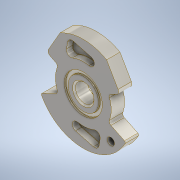
# Autodesk Inventor part: Part005. Frontal Faucet Core
Saved by Autodesk Inventor 2022.2 (Build 262287010, 287A)
## iProperties
Created: 2022-11-29
Part Number: Part005. Frontal Faucet Core
Material: Stainless Steel
Document SubType Name: Modeling
Designer: User
Mass: 160.563 g
Surface Area: 77.5804 cm^2
Volume: 20.0704 cm^3
Density: 8 g/cm^3
Appearance: Titanium - Polished
Author: User
Autodesk Inventor part; units mm, degrees
ref_plane "YZ Plane" through (0, 0, 0) normal (1, 0, 0) x (0, 1, 0)
ref_plane "XZ Plane" through (0, 0, 0) normal (0, 1, 0) x (-1, 0, 0)
sketch "Sketch1" plane through (0, 0, 0) normal (0, 0, 1) x (1, 0, 0)
  arc A0 (-28.473878, -15.0359) -> (28.473878, -15.0359) centre (0, 0) ccw
  arc A1 (-17.077087, -8.329052) -> (-17.077087, 8.329052) centre (0, 0) ccw construction
  line L0 (-18.788881, 9.163949) -> (-22.595928, 11.02077)
  line L1 (-23.665064, 14.517756) -> (-15.871417, 28.016747)
  line L2 (-18.788881, -9.163949) -> (-28.027967, -13.670153)
  arc A2 (-15.871417, 28.016747) -> (-28.941168, -14.115551) centre (0, 0) ccw construction
  arc A3 (-17.792706, 6.664803) -> (-17.792706, -6.664803) centre (0, 0) ccw
  line L3 (0, -45.08) -> (0, 45.08) construction
  line L4 (-69.758488, 0) -> (68.933664, 0) construction
  arc A4 (-17.792706, 6.664803) -> (-18.788881, 9.163949) centre (-19.665623, 7.366361) ccw
  arc A5 (-18.788881, -9.163949) -> (-17.792706, -6.664803) centre (-19.665623, -7.366361) ccw
  arc A6 (-28.027967, -13.670153) -> (-28.473878, -15.0359) centre (-27.589596, -14.568947) ccw
  arc A7 (-23.665064, 14.517756) -> (-22.595928, 11.02077) centre (-21.5, 13.267756) ccw
  arc A8 (17.077087, 8.329052) -> (17.077087, -8.329052) centre (0, 0) ccw construction
  line L5 (18.788881, 9.163949) -> (22.595928, 11.02077)
  line L6 (23.665064, 14.517756) -> (15.871417, 28.016747)
  line L7 (18.788881, -9.163949) -> (28.027967, -13.670153)
  arc A9 (28.941168, -14.115551) -> (32.2, 0) centre (0, 0) ccw construction
  arc A10 (17.792706, -6.664803) -> (17.792706, 6.664803) centre (0, 0) ccw
  line L8 (69.758488, 0) -> (-68.933664, 0) construction
  arc A11 (18.788881, 9.163949) -> (17.792706, 6.664803) centre (19.665623, 7.366361) ccw
  arc A12 (17.792706, -6.664803) -> (18.788881, -9.163949) centre (19.665623, -7.366361) ccw
  arc A13 (28.473878, -15.0359) -> (28.027967, -13.670153) centre (27.589596, -14.568947) ccw
  arc A14 (22.595928, 11.02077) -> (23.665064, 14.517756) centre (21.5, 13.267756) ccw
  arc A15 (32.2, 0) -> (15.871417, 28.016747) centre (0, 0) ccw construction
  arc A16 (32.2, 0) -> (15.871417, 28.016747) centre (0, 0) ccw construction
  arc A17 (28.473878, -15.0359) -> (32.2, 0) centre (0, 0) ccw construction
  arc A18 (15.871417, 28.016747) -> (-15.871417, 28.016747) centre (0, 0) ccw
  circle A19 centre (0, 0) radius 6.3
  dimension "d0" = 64.4
  dimension "d1" = 38
  dimension "d2" = 26
  dimension "d3" = 52
  dimension "d4" = 30
  dimension "d5" = 2
  dimension "d6" = 1
  dimension "d7" = 2.5
  dimension "d8" = 48
  dimension "d9" = 12.6
  constraints: 43 point on circle, 20 centre point, 18 symmetric about line, 14 end point, 9 point on line, 8 tangent, 4 coincident, 1 equal radius, 7 other
  measures "d0" diameter of A0
  measures "d1" diameter of A1
  measures "d2" angle of L4 L2
  measures "d3" angle of L2 L0
  measures "d4" angle of L3 L1
  measures "d5" radius of A4
  measures "d6" radius of A6
  measures "d7" radius of A7
  measures "d9" diameter of A19
extrude "Extrusion1" add sketch "Sketch1" along normal blind 9.1
sketch "Sketch2" plane through (0, 0, 9.1) normal (0, 0, 1) x (1, 0, 0)
  arc A0 (-28.027967, -13.670153) -> (-28.473878, -15.0359) centre (-27.589596, -14.568947) ccw
  arc A1 (-28.473878, -15.0359) -> (28.473878, -15.0359) centre (0, 0) ccw
  arc A2 (28.473878, -15.0359) -> (28.027967, -13.670153) centre (27.589596, -14.568947) ccw
  line L0 (28.027967, -13.670153) -> (18.788881, -9.163949)
  arc A3 (17.792706, -6.664803) -> (18.788881, -9.163949) centre (19.665623, -7.366361) ccw
  arc A4 (17.792706, -6.664803) -> (17.792706, 6.664803) centre (0, 0) ccw
  arc A5 (18.788881, 9.163949) -> (17.792706, 6.664803) centre (19.665623, 7.366361) ccw
  line L1 (18.788881, 9.163949) -> (22.595928, 11.02077)
  arc A6 (22.595928, 11.02077) -> (23.665064, 14.517756) centre (21.5, 13.267756) ccw
  line L2 (23.665064, 14.517756) -> (15.871417, 28.016747)
  arc A7 (15.871417, 28.016747) -> (-15.871417, 28.016747) centre (0, 0) ccw
  line L3 (-15.871417, 28.016747) -> (-23.665064, 14.517756)
  arc A8 (-23.665064, 14.517756) -> (-22.595928, 11.02077) centre (-21.5, 13.267756) ccw
  line L4 (-22.595928, 11.02077) -> (-18.788881, 9.163949)
  arc A9 (-17.792706, 6.664803) -> (-18.788881, 9.163949) centre (-19.665623, 7.366361) ccw
  arc A10 (-17.792706, 6.664803) -> (-17.792706, -6.664803) centre (0, 0) ccw
  arc A11 (-18.788881, -9.163949) -> (-17.792706, -6.664803) centre (-19.665623, -7.366361) ccw
  line L5 (-18.788881, -9.163949) -> (-28.027967, -13.670153)
  circle A12 centre (0, 0) radius 6.3
  arc A13 (17.792706, 6.664803) -> (3.886364, 18.598284) centre (0, 0) ccw construction
  arc A14 (-11.454423, 20.812568) -> (-7.340909, 17.524584) centre (-8.5, 20.291624) ccw
  arc A15 (3.886364, 18.598284) -> (5.276457, 24.432633) centre (4.5, 21.534855) ccw
  line L6 (0, -45.08) -> (0, 45.08) construction
  line L7 (-11.454423, 20.812568) -> (-10.658601, 25.3259)
  line L8 (-6.927721, 27.702733) -> (5.276457, 24.432633)
  arc A16 (-6.927721, 27.702733) -> (-10.658601, 25.3259) centre (-7.704178, 24.804955) ccw
  arc A17 (-7.340909, 17.524584) -> (-17.792706, 6.664803) centre (0, 0) ccw construction
  arc A18 (3.886364, 18.598284) -> (-7.340909, 17.524584) centre (0, 0) ccw
  arc A19 (6.927721, -27.702733) -> (10.658601, -25.3259) centre (7.704178, -24.804955) ccw
  arc A20 (7.340909, -17.524584) -> (17.792706, -6.664803) centre (0, 0) ccw construction
  arc A21 (-17.792706, -6.664803) -> (-3.886364, -18.598284) centre (0, 0) ccw construction
  arc A22 (-3.886364, -18.598284) -> (7.340909, -17.524584) centre (0, 0) ccw
  arc A23 (11.454423, -20.812568) -> (7.340909, -17.524584) centre (8.5, -20.291624) ccw
  arc A24 (-3.886364, -18.598284) -> (-5.276457, -24.432633) centre (-4.5, -21.534855) ccw
  line L9 (11.454423, -20.812568) -> (10.658601, -25.3259)
  line L10 (6.927721, -27.702733) -> (-5.276457, -24.432633)
  dimension "d12" = 6
  dimension "d13" = 11.5
  dimension "d14" = 13
  dimension "d15" = 3
  dimension "d16" = 10
  dimension "d20" = 360
  constraints: 24 point on circle, 12 centre point, 8 end point, 6 tangent, 1 coincident, 1 equal radius, 41 other
  measures "d12" diameter of A14
  measures "d14" horizontal distance of A15.centre A14.centre
  measures "d15" radius of A16
  measures "d16" angle of L6 L7
extrude "Extrusion2" cut sketch "Sketch2" against normal blind 4.3 contours L7 A16 L8 A15 A18 A14 | L10 A24 A22 A23 L9 A19
fillet "Fillet1" radius 0.2 12 edges at (-10.3731, 17.9482, 4.8) (-11.0565, 23.0692, 4.8) (-9.3161, 27.3351, 4.8) (-0.8256, 26.0677, 4.8) (7.4183, 20.8395, 4.8) (-1.8088, 18.9137, 4.8) (-7.4183, -20.8395, 4.8) (1.8088, -18.9137, 4.8) (10.3731, -17.9482, 4.8) (11.0565, -23.0692, 4.8) (9.3161, -27.3351, 4.8) (0.8256, -26.0677, 4.8)
sketch "Sketch3" plane through (0, 0, 9.1) normal (0, 0, 1) x (1, 0, 0)
  arc A0 (6.927721, -27.702733) -> (10.658601, -25.3259) centre (7.704178, -24.804955) ccw
  line L0 (6.927721, -27.702733) -> (-5.276457, -24.432633)
  arc A1 (-3.886364, -18.598284) -> (-5.276457, -24.432633) centre (-4.5, -21.534855) ccw
  arc A2 (-3.886364, -18.598284) -> (7.340909, -17.524584) centre (0, 0) ccw
  arc A3 (11.454423, -20.812568) -> (7.340909, -17.524584) centre (8.5, -20.291624) ccw
  line L1 (11.454423, -20.812568) -> (10.658601, -25.3259)
  arc A4 (-11.454423, 20.812568) -> (-7.340909, 17.524584) centre (-8.5, 20.291624) ccw
  line L2 (-11.454423, 20.812568) -> (-10.658601, 25.3259)
  arc A5 (-6.927721, 27.702733) -> (-10.658601, 25.3259) centre (-7.704178, 24.804955) ccw
  line L3 (-6.927721, 27.702733) -> (5.276457, 24.432633)
  arc A6 (3.886364, 18.598284) -> (5.276457, 24.432633) centre (4.5, 21.534855) ccw
  arc A7 (3.886364, 18.598284) -> (-7.340909, 17.524584) centre (0, 0) ccw
  arc A8 (-28.027967, -13.670153) -> (-28.473878, -15.0359) centre (-27.589596, -14.568947) ccw
  arc A9 (-28.473878, -15.0359) -> (28.473878, -15.0359) centre (0, 0) ccw
  arc A10 (28.473878, -15.0359) -> (28.027967, -13.670153) centre (27.589596, -14.568947) ccw
  line L4 (28.027967, -13.670153) -> (18.788881, -9.163949)
  arc A11 (17.792706, -6.664803) -> (18.788881, -9.163949) centre (19.665623, -7.366361) ccw
  arc A12 (17.792706, -6.664803) -> (17.792706, 6.664803) centre (0, 0) ccw
  arc A13 (18.788881, 9.163949) -> (17.792706, 6.664803) centre (19.665623, 7.366361) ccw
  line L5 (18.788881, 9.163949) -> (22.595928, 11.02077)
  arc A14 (22.595928, 11.02077) -> (23.665064, 14.517756) centre (21.5, 13.267756) ccw
  line L6 (23.665064, 14.517756) -> (15.871417, 28.016747)
  arc A15 (15.871417, 28.016747) -> (-15.871417, 28.016747) centre (0, 0) ccw
  line L7 (-15.871417, 28.016747) -> (-23.665064, 14.517756)
  arc A16 (-23.665064, 14.517756) -> (-22.595928, 11.02077) centre (-21.5, 13.267756) ccw
  line L8 (-22.595928, 11.02077) -> (-18.788881, 9.163949)
  arc A17 (-17.792706, 6.664803) -> (-18.788881, 9.163949) centre (-19.665623, 7.366361) ccw
  arc A18 (-17.792706, 6.664803) -> (-17.792706, -6.664803) centre (0, 0) ccw
  arc A19 (-18.788881, -9.163949) -> (-17.792706, -6.664803) centre (-19.665623, -7.366361) ccw
  line L9 (-18.788881, -9.163949) -> (-28.027967, -13.670153)
  circle A20 centre (0, 0) radius 6.3
  circle A21 centre (0, 0) radius 10.4
  circle A22 centre (0, 0) radius 12.9
  dimension "d25" = 20.8
  dimension "d26" = 25.8
  constraints: 2 centre point, 2 coincident
  measures "d25" diameter of A21
  measures "d26" diameter of A22
extrude "Extrusion3" cut sketch "Sketch3" against normal blind 1 contours A22
fillet "Fillet2" radius 0.2 2 edges at (-12.9, 0, 8.1) (-10.4, 0, 8.1)
ref_plane "Work Plane1" through (0, 0, 0.7) normal (0, 0, -1) x (-1, 0, 0)
sketch "Sketch4" plane through (0, 0, 0.7) normal (0, 0, -1) x (-1, 0, 0)
  arc A0 (-10.695652, -17.488654) -> (10.695652, -17.488654) centre (0, 0) ccw
  arc A1 (-10.886228, -22.782725) -> (10.886228, -22.782725) centre (0, 0) ccw
  line L0 (-11, 22.602268) -> (-11, 17.659275)
  line L1 (0, -45.08) -> (0, 45.08) construction
  line L2 (11, 22.602268) -> (11, 17.659275)
  arc A2 (-11, 22.728011) -> (-11, -22.728011) centre (0, 0) ccw construction
  arc A3 (-11, 17.298844) -> (-11, -17.298844) centre (0, 0) ccw construction
  line L3 (-11, 17.298844) -> (-11, -22.602268) construction
  line L4 (11, 17.298844) -> (11, -17.298844) construction
  arc A4 (10.695652, 17.488654) -> (-10.695652, 17.488654) centre (0, 0) ccw
  arc A5 (11, -17.298844) -> (11, 17.298844) centre (0, 0) ccw construction
  arc A6 (10.886228, 22.782725) -> (-10.886228, 22.782725) centre (0, 0) ccw
  arc A7 (11, -22.728011) -> (11, 22.728011) centre (0, 0) ccw construction
  line L5 (11, -17.659275) -> (11, -22.602268)
  line L6 (-11, -17.659275) -> (-11, -22.728011)
  arc A8 (-10.886228, 22.782725) -> (-11, 22.602268) centre (-10.8, 22.602268) ccw
  arc A9 (-10.695652, -17.488654) -> (-11, -17.659275) centre (-10.8, -17.659275) ccw
  arc A10 (-11, -22.602268) -> (-10.886228, -22.782725) centre (-10.8, -22.602268) ccw
  arc A11 (10.886228, -22.782725) -> (11, -22.602268) centre (10.8, -22.602268) ccw
  arc A12 (11, -17.659275) -> (10.695652, -17.488654) centre (10.8, -17.659275) ccw
  arc A13 (11, 22.602268) -> (10.886228, 22.782725) centre (10.8, 22.602268) ccw
  arc A14 (10.695652, 17.488654) -> (11, 17.659275) centre (10.8, 17.659275) ccw
  arc A15 (-11, 17.659275) -> (-10.695652, 17.488654) centre (-10.8, 17.659275) ccw
  dimension "d31" = 41
  dimension "d32" = 50.5
  dimension "d33" = 22
  dimension "d34" = 0.2
  constraints: 41 point on circle, 16 centre point, 16 tangent, 12 end point, 10 point on line, 7 equal radius, 3 vertical, 2 coincident, 2 symmetric about line, 1 collinear
  measures "d31" diameter of A0
  measures "d32" diameter of A1
  measures "d33" distance between parallel lines of L2 L0
  measures "d34" radius of A8
extrude "Extrusion4" cut sketch "Sketch4" along normal blind 1 draft 60
chamfer "Chamfer1" distance 0.2 angle 45 1 edges at (-6.3, 0, 0)
chamfer "Chamfer2" distance 1 angle 45 1 edges at (-6.3, 0, 9.1)
sketch "Sketch5" plane through (0, 0, 9.1) normal (0, 0, 1) x (1, 0, 0)
  arc A0 (-28.027967, -13.670153) -> (-28.473878, -15.0359) centre (-27.589596, -14.568947) ccw
  arc A1 (-28.473878, -15.0359) -> (28.473878, -15.0359) centre (0, 0) ccw
  arc A2 (28.473878, -15.0359) -> (28.027967, -13.670153) centre (27.589596, -14.568947) ccw
  line L0 (28.027967, -13.670153) -> (18.788881, -9.163949)
  arc A3 (17.792706, -6.664803) -> (18.788881, -9.163949) centre (19.665623, -7.366361) ccw
  arc A4 (17.792706, -6.664803) -> (17.792706, 6.664803) centre (0, 0) ccw
  arc A5 (18.788881, 9.163949) -> (17.792706, 6.664803) centre (19.665623, 7.366361) ccw
  line L1 (18.788881, 9.163949) -> (22.595928, 11.02077)
  arc A6 (22.595928, 11.02077) -> (23.665064, 14.517756) centre (21.5, 13.267756) ccw
  line L2 (23.665064, 14.517756) -> (15.871417, 28.016747)
  arc A7 (15.871417, 28.016747) -> (-15.871417, 28.016747) centre (0, 0) ccw
  line L3 (-15.871417, 28.016747) -> (-23.665064, 14.517756)
  arc A8 (-23.665064, 14.517756) -> (-22.595928, 11.02077) centre (-21.5, 13.267756) ccw
  line L4 (-22.595928, 11.02077) -> (-18.788881, 9.163949)
  arc A9 (-17.792706, 6.664803) -> (-18.788881, 9.163949) centre (-19.665623, 7.366361) ccw
  arc A10 (-17.792706, 6.664803) -> (-17.792706, -6.664803) centre (0, 0) ccw
  arc A11 (-18.788881, -9.163949) -> (-17.792706, -6.664803) centre (-19.665623, -7.366361) ccw
  line L5 (-18.788881, -9.163949) -> (-28.027967, -13.670153)
  arc A12 (-11.454423, 20.812568) -> (-7.340909, 17.524584) centre (-8.5, 20.291624) ccw
  line L6 (-11.454423, 20.812568) -> (-10.658601, 25.3259)
  arc A13 (-6.927721, 27.702733) -> (-10.658601, 25.3259) centre (-7.704178, 24.804955) ccw
  line L7 (-6.927721, 27.702733) -> (5.276457, 24.432633)
  arc A14 (3.886364, 18.598284) -> (5.276457, 24.432633) centre (4.5, 21.534855) ccw
  arc A15 (3.886364, 18.598284) -> (-7.340909, 17.524584) centre (0, 0) ccw
  arc A16 (6.927721, -27.702733) -> (10.658601, -25.3259) centre (7.704178, -24.804955) ccw
  line L8 (6.927721, -27.702733) -> (-5.276457, -24.432633)
  arc A17 (-3.886364, -18.598284) -> (-5.276457, -24.432633) centre (-4.5, -21.534855) ccw
  arc A18 (-3.886364, -18.598284) -> (7.340909, -17.524584) centre (0, 0) ccw
  arc A19 (11.454423, -20.812568) -> (7.340909, -17.524584) centre (8.5, -20.291624) ccw
  line L9 (11.454423, -20.812568) -> (10.658601, -25.3259)
  circle A20 centre (0, 0) radius 12.9
  line L10 (-40.268433, 0) -> (40.268433, 0) construction
  line L11 (0, 0) -> (18.73833, -18.73833) construction
  dimension "d43" = 45
  dimension "d44" = 26.5
  constraints: 2 end point
  measures "d43" angle of L10 L11
  measures "d44" distance of point (0, 0) L11.end
hole "Hole1" at (18.73833, -18.73833, 9.1) direction (0, 0, -1) diameter 5 end through all
body "Solid1"
